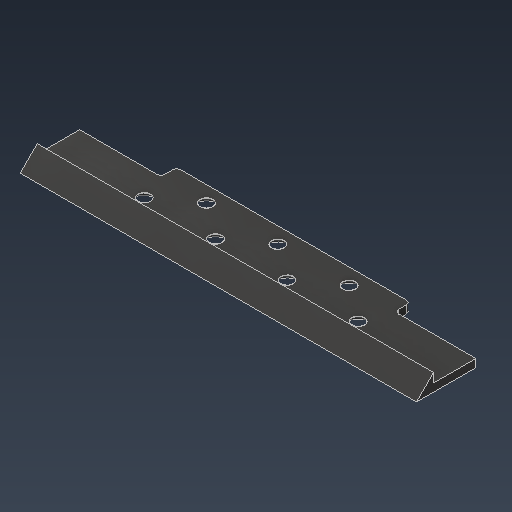
# Autodesk Inventor part: Plog2
Saved by Autodesk Inventor 2027.1 (Build 311270010, 270A)
## iProperties
Created: 2022-01-27
Part Number: Plog2
Material: Steel, Carbon
Document SubType Name: Modeling
Designer: Michał
Density: 7.85 g/cm^3
Appearance: Dark Gray
Mass: 32.9087 g
Surface Area: 43.2545 cm^2
Volume: 4.19219 cm^3
Author: Michał
Autodesk Inventor part; units mm, degrees
ref_plane "YZ Plane" through (0, 0, 0) normal (1, 0, 0) x (0, 1, 0)
ref_plane "XZ Plane" through (0, 0, 0) normal (0, 1, 0) x (-1, 0, 0)
ref_plane "XY Plane" through (0, 0, 0) normal (0, 0, 1) x (1, 0, 0)
sketch "Szkic1" plane through (0, 0, 0) normal (1, 0, 0) x (0, 1, 0)
  line L0 (0, 0) -> (2, -2)
  line L1 (2, -2) -> (2, -19)
  line L2 (2, -19) -> (0, -19)
  line L3 (0, -19) -> (0, -2)
  line L4 (0, -2) -> (0, 0)
  line L5 (0, -2) -> (2, -2)
  line L6 (2, -2) -> (4.3, -4.3)
  line L7 (4.3, -4.3) -> (2, -4.3)
  line L8 (2, -2) -> (4.3, -4.3)
  line L9 (4.3, -4.3) -> (2, -4.3)
  line L10 (4, -4) -> (4, -4.3) construction
  line L11 (4, -4) -> (2, -4) construction
  line L12 (4.3, -4.3) -> (4.3, -4.8)
  line L13 (4.3, -4.8) -> (2, -4.8)
  line L14 (0, 0) -> (-0.5, 0)
  line L15 (-0.5, 0) -> (-0.5, -19)
  line L16 (-0.5, -19) -> (0, -19)
  line L17 (0, -19) -> (0, 0)
  point P0 (5, -5)
  point P1 (4.3, -4.3)
  dimension "d1" = 2
  dimension "d2" = 45
  dimension "d44" = 45
  dimension "d45" = 2
  dimension "d46" = 17
  dimension "d50" = -4.3
  dimension "d51" = 19
  dimension "d54" = 0
  dimension "d98" = 2.3
  dimension "d125" = 4
  dimension "d126" = 0.3
  dimension "d156" = 0.5
  dimension "d157" = 0.5
  constraints: 36 end point, 10 point on line, 9 perpendicular, 2 horizontal, 2 parallel, 2 vertical, 1 coincident, 2 other
  measures "d1" distance between parallel lines of L4 L1
  measures "d2" angle of L4 L0
  measures "d44" angle of L7 L6
  measures "d45" distance of L3.end L0.start
  measures "d46" distance of L2.end L3.end
  measures "d51" distance from line of L2 L0.start
  measures "d98" distance from line of L1 L6.end
  measures "d125" distance between parallel lines of L3 L10
  measures "d126" distance between parallel lines of L7 L11
  measures "d156" distance of L12.start L12.end
  measures "d157" distance between parallel lines of L15 L4
extrude "Wyciągnięcie proste1" add sketch "Szkic1" along normal mid plane 100 contours L0 L5 L4 | L6 L7 L1 | L1 L2 L3 L5
sketch "Sketch4" plane through (-50, 0, -19) normal (0, -1, 0) x (1, 0, 0)
  line L0 (0, 0) -> (0, 19) projected
  line L1 (0, 0) -> (100, 0) projected
  line L2 (100, 19) -> (100, 0) projected
  line L3 (100, 19) -> (0, 19) projected
  line L4 (80, 0) -> (80, 19)
  line L5 (100, 19) -> (50, 19) projected
  line L6 (20, 19) -> (20, 0)
  line L7 (0, 0) -> (100, 0) projected
  line L8 (0, 14.7) -> (100, 14.7) projected
  circle A0 centre (77, 10.7) radius 3
  circle A1 centre (41, 10.7) radius 3
  circle A2 centre (23, 10.7) radius 3
  line L9 (80, 10.7) -> (20, 10.7)
  line L10 (80, 4) -> (20, 4)
  circle A3 centre (59, 10.7) radius 3
  circle A4 centre (68, 4) radius 3
  circle A5 centre (50, 4) radius 3
  circle A6 centre (32, 4) radius 3
  dimension "d67" = 6
  dimension "d70" = 6
  dimension "d22" = 20
  dimension "d23" = 20
  dimension "d69" = 6
  dimension "d75" = 18
  dimension "d127" = 6
  dimension "d129" = 18
  dimension "d139" = 18
  dimension "d140" = 6
  dimension "d141" = 6
  dimension "d142" = 6
  dimension "d143" = 9
  dimension "d144" = 9
  dimension "d145" = 9
  dimension "d146" = 9
  dimension "d147" = 9
  dimension "d148" = 9
  dimension "d149" = 4
  dimension "d150" = 4
  constraints: 11 point on line, 8 end point, 5 centre point, 2 horizontal, 2 horizontal alignment, 2 perpendicular, 2 vertical, 1 midpoint, 4 other
  measures "d22" distance between parallel lines of L2 L4
  measures "d23" distance between parallel lines of L0 L6
  measures "d69" diameter of A1
  measures "d75" distance of point (23, 10.7) A1.centre
  measures "d127" diameter of A3
  measures "d129" distance of A3.centre A1.centre
  measures "d139" distance of point (77, 10.7) A3.centre
  measures "d140" diameter of A4
  measures "d141" diameter of A5
  measures "d142" diameter of A6
  measures "d143" horizontal distance of A6.centre point (23, 10.7)
  measures "d144" horizontal distance of A6.centre A1.centre
  measures "d145" horizontal distance of A5.centre A1.centre
  measures "d146" horizontal distance of A5.centre A3.centre
  measures "d147" horizontal distance of A4.centre A3.centre
  measures "d148" horizontal distance of A4.centre point (77, 10.7)
  measures "d149" distance between parallel lines of L1 L10
  measures "d150" distance between parallel lines of L8 L9
hole "Hole2" at (27, 0, -8.3) at (-9, 0, -8.3) at (-27, 0, -8.3) at (9, 0, -8.3) at (0, 0, -15) at (18, 0, -15) at (-18, 0, -15) direction (0, 1, 0) diameter 3.2 depth 8.8 countersink diameter 7 countersink angle 90 clearance for "Countersunk Flat Head Screw ISO 2009/7046" size "M3" standard "ISO"
extrude "Extrusion7" [suppressed]
sketch "Sketch5" plane through (-50, 0, 0) normal (0, -1, 0) x (1, 0, 0)
  line L0 (100, 0) -> (100, -19) projected
  line L1 (100, 0) -> (0, 0) projected
  line L2 (0, -19) -> (0, 0) projected
  line L3 (100, -15) -> (79.5, -15)
  line L4 (79.5, -15) -> (79.5, -32.132)
  line L5 (79.5, -32.132) -> (100, -32.132)
  line L6 (100, -32.132) -> (100, -15)
  line L7 (0, -19) -> (20.5, -19)
  line L8 (20.5, -19) -> (20.5, -15)
  line L9 (20.5, -15) -> (0, -15)
  line L10 (0, -15) -> (0, -19)
  circle A0 centre (23, -8.3) radius 3.5 projected
  circle A1 centre (41, -8.3) radius 3.5 projected
  circle A2 centre (77, -8.3) radius 3.5 projected
  line L11 (0, -19) -> (100, -19) projected
  point P0 (50, 0)
  point P1 (0, -15)
  point P2 (100, -30)
  dimension "d55" = 20.5
  dimension "d56" = 20.5
  dimension "d61" = 15
  dimension "d62" = 15
  constraints: 16 end point, 4 parallel, 2 horizontal, 2 perpendicular, 1 point on line
  measures "d55" distance of L8.end L9.end
  measures "d56" distance of L3.start L3.end
  measures "d61" distance between parallel lines of L1 L9
  measures "d62" distance between parallel lines of L1 L3
extrude "Extrusion5" cut sketch "Sketch5" along normal through all both and the other way through all contours L0 L11 L4 L3 | L6 L5 L4 L11 | L9 L8 L7 L2
fillet "Fillet2" radius 1 2 edges at (-29.5, 1, -19) (29.5, 1, -19)
fillet "Fillet3" radius 1 2 edges at (-29.5, 1, -15) (29.5, 1, -15)
sketch "Sketch10" plane through (50, 0, 0) normal (1, 0, 0) x (0, 0, -1)
  line L0 (30.7582, 13.788) -> (30.3919, 3.2994) projected
  line L1 (30.5751, 8.5437) -> (-8.4118, 9.9052)
  line L2 (15, 0) -> (15, 2) projected
  line L3 (15, 2) -> (4.3, 2) projected
  line L4 (4.3, 2) -> (4.3, 4.3) projected
  line L5 (4.3, 4.3) -> (0, 0) projected
  line L6 (0, 0) -> (15, 0) projected
  line L7 (4.3, 2) -> (15, 2) projected
  line L8 (4.3, 2) -> (3.8, 2)
  circle A0 centre (63.2278, 12.35) radius 15 projected
  line L9 (63.2278, 12.35) -> (63.2278, -2.65)
  line L10 (63.2278, -2.65) -> (0, 0)
  line L11 (0, 0) -> (0.1802, 4.3)
  line L12 (0.1802, 4.3) -> (3.8, 4.3)
  line L13 (3.8, 4.3) -> (3.8, 2)
  line L14 (3.8, 4.3) -> (4.3, 4.3) construction
  point P0 (3.8, 3.8)
  dimension "d166" = 90
  dimension "d167" = 0.5
  constraints: 16 end point, 2 perpendicular, 1 collinear, 1 horizontal, 1 midpoint, 1 point on line, 1 vertical, 1 vertical alignment, 1 other
  measures "d166" angle of L0 L1
  measures "d167" distance of L3.end L8.end
extrude "Extrusion9" [suppressed]
sketch "Sketch11" plane through (50, 0, 0) normal (1, 0, 0) x (0, 0, -1)
  line L0 (3.8, 4.3) -> (3.8, 2) projected
  line L1 (4.3, 2) -> (3.8, 2) projected
  line L2 (4.3, 2) -> (4.3, 4.3) projected
  line L3 (4.3, 4.3) -> (0, 0) projected
  point P0 (3.8, 3.8)
extrude "Extrusion10" [suppressed]
sketch "Sketch12" plane through (-28.5, 0, -19) normal (0, -1, 0) x (1, 0, 0)
  arc A0 (57, 0) -> (58, 1) centre (57, 1) ccw projected
  line L0 (58, 1) -> (58, 3) projected
  arc A1 (59, 4) -> (58, 3) centre (59, 3) ccw projected
  line L1 (59, 4) -> (78.5, 4) projected
  line L2 (78.5, 19) -> (78.5, 4) projected
  line L3 (78.5, 19) -> (-21.5, 19) projected
  line L4 (-21.5, 4) -> (-21.5, 19) projected
  line L5 (-21.5, 4) -> (-2, 4) projected
  arc A2 (-1, 3) -> (-2, 4) centre (-2, 3) ccw projected
  line L6 (-1, 3) -> (-1, 1) projected
  arc A3 (-1, 1) -> (0, 0) centre (0, 1) ccw projected
  line L7 (0, 0) -> (57, 0) projected
  circle A4 centre (55.5, 10.7) radius 3.5 projected
  circle A5 centre (19.5, 10.7) radius 3.5 projected
  circle A6 centre (1.5, 10.7) radius 3.5 projected
  circle A7 centre (37.5, 10.7) radius 3.5 projected
  circle A8 centre (28.5, 4) radius 3.5 projected
  circle A9 centre (46.5, 4) radius 3.5 projected
  circle A10 centre (10.5, 4) radius 3.5 projected
  arc A11 (57, 0.5) -> (57.5, 1) centre (57, 1) ccw
  line L8 (57.5, 1) -> (57.5, 3)
  arc A12 (59, 4.5) -> (57.5, 3) centre (59, 3) ccw
  line L9 (59, 4.5) -> (78, 4.5)
  line L10 (78, 4.5) -> (78, 18.5)
  line L11 (78, 18.5) -> (-21, 18.5)
  line L12 (-21, 18.5) -> (-21, 4.5)
  line L13 (-21, 4.5) -> (-2, 4.5)
  arc A13 (-0.5, 3) -> (-2, 4.5) centre (-2, 3) ccw
  line L14 (-0.5, 3) -> (-0.5, 1)
  arc A14 (-0.5, 1) -> (0, 0.5) centre (0, 1) ccw
  line L15 (0, 0.5) -> (57, 0.5)
  line L16 (57, 0.5) -> (57.866, 0.5)
  line L17 (0, 0.5) -> (-0.866, 0.5)
  point P0 (28.5, 19)
  dimension "d172" = 0.5
  constraints: 20 end point, 10 point on circle, 4 centre point, 1 perpendicular, 1 point on line, 1 tangent, 11 other
  measures "d172" distance between parallel lines of L7 L15
extrude "Extrusion11" [suppressed]
fillet "Fillet4" [suppressed]
equation "\"d23\" = d22"
equation "\"d56\" = d55"
equation "\"d62\" = d61"
equation "\"d64\" = d80"
equation "\"d79\" = d64"
equation "\"d80\" = 4.648267"
